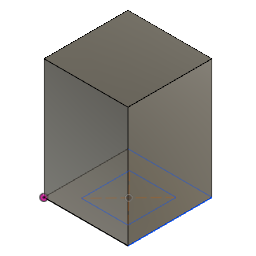
building (Autodesk Fusion 360 design; units mm, degrees)
Autodesk Fusion 360 part; units mm, degrees
sketch "Sketch1" plane through (0, 0, 0) normal (0, 0, 1) x (1, 0, 0)
  line L0 (0, 0) -> (14, 0)
  line L1 (14, 0) -> (14, 14)
  line L2 (14, 14) -> (0, 14)
  line L3 (0, 14) -> (0, 0)
  line L4 (11, 11) -> (3.2653, 11)
  line L5 (3.2653, 11) -> (3.2653, 2.9996)
  line L6 (3.2653, 2.9996) -> (11, 2.9996)
  line L7 (11, 2.9996) -> (11, 11)
  line L8 (11, 11) -> (3.2653, 2.9996) construction
  line L9 (3.2653, 11) -> (11, 2.9996) construction
  point P0 (7.1326, 6.9998)
  constraint horizontal L0
  constraint vertical L1
  constraint horizontal L2
  constraint vertical L3
  constraint coincident L0.start L3.end
  constraint perpendicular L4 L5
  constraint parallel L4 L6
  constraint parallel L5 L7
  constraint horizontal L4
  constraint coincident L8 P0
  constraint coincident L9 P0
extrude "Extrude1" add sketch "Sketch1" along normal blind 20 contours L0 L1 L2 L3 | L4 L5 L6 L7
extrude "Extrude2" cut sketch "Sketch1" along normal blind 19 contours L4 L5 L6 L7
